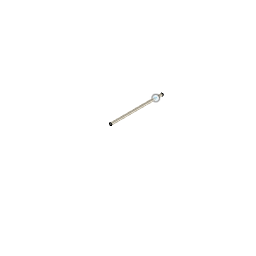
Long Bolt Between Wheels (Autodesk Fusion 360 design; units mm, degrees)
Autodesk Fusion 360 part; units mm, degrees
sketch "Holes" plane through (0, 35, 0) normal (0, 1, 0) x (-1, 0, 0)
  circle A0 centre (-31, 17.1) radius 1
extrude "Extrude1" add sketch "Holes" along normal blind 2.2 and the other way blind 23
extrude "Extrude2" add 1 faces at (30.6704, 12, 16.7741) along direction (0, -1, 0) blind 13
extrude "Extrude3" add 1 faces at (30.6704, -1, 16.7741) along direction (0, -1, 0) blind 2
extrude "Extrude4" add 1 faces at (30.6704, 37.2, 16.7741) along direction (0, 1, 0) blind 3
named bodies: "Base"
